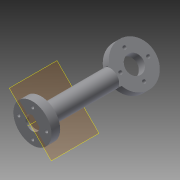
# Autodesk Inventor part: neck_v2
Saved by Autodesk Inventor 2014 (Build 180170000, 170)
## iProperties
Created: 2014-01-09
Part Number: neck_v2
Material: Générique
Document SubType Name: Modeling
Designer: helly
Density: 1 g/cm^3
Appearance: Par défaut
Author: helly
Autodesk Inventor part; units mm, degrees
ref_plane "YZ Plane" through (0, 0, 0) normal (1, 0, 0) x (0, 1, 0)
ref_plane "XZ Plane" through (0, 0, 0) normal (0, 1, 0) x (-1, 0, 0)
sketch "Esquisse1" plane through (0, 0, 0) normal (0, 1, 0) x (-1, 0, 0)
  circle A0 centre (0, 0) radius 11
  line L0 (0, 0) -> (-8, 0) construction
  circle A1 centre (-8, 0) radius 1
  circle A2 centre (0, -8) radius 1
  circle A3 centre (8, 0) radius 1
  circle A4 centre (0, 8) radius 1
  circle A5 centre (0, 0) radius 4
  dimension "d0" = 22
  dimension "d1" = 8
  dimension "d2" = 2
  dimension "d5" = 360
  dimension "d7" = 8
  constraints: 6 centre point, 5 coincident, 2 end point, 1 horizontal, 11 other
  measures "d0" diameter of A0
  measures "d1" distance of L0.start L0.end
  measures "d2" diameter of A1
  measures "d7" diameter of A5
extrude "Extrusion1" add sketch "Esquisse1" along normal blind 5
sketch "Esquisse2" plane through (0, 5, 0) normal (0, 1, 0) x (1, 0, 0)
  circle A0 centre (0, 0) radius 4 projected
extrude "Extrusion2" add sketch "Esquisse2" against normal blind 3
sketch "Esquisse3" plane through (0, 5, 0) normal (0, 1, 0) x (1, 0, 0)
  circle A0 centre (0, 0) radius 11 projected
  circle A1 centre (0, 0) radius 5
  dimension "d12" = 10
  constraints: 1 centre point, 1 coincident
  measures "d12" diameter of A1
extrude "Extrusion3" add sketch "Esquisse3" along normal blind 40 contours A1
ref_plane "Plan de construction1" through (0, 0, 0) normal (0.7071, 0, 0.7071) x (0, 1, 0)
sketch "Esquisse4" plane through (0, 0, 0) normal (0.7071, 0, 0.7071) x (0, 1, 0)
  line L0 (0, 0) -> (5, 0) construction
  line L1 (5, 0) -> (5, -5) construction
  line L2 (5, 0) -> (5, 5)
  line L3 (5, 0) -> (5, -5)
  line L4 (0, 0) -> (45, 0) construction
  line L5 (45, 0) -> (57, 0) construction
  circle A0 centre (57, 0) radius 12
  circle A1 centre (57, 0) radius 8 construction
  line L6 (0, 0) -> (45, 0) construction
  line L7 (45, 0) -> (57, 0) construction
  circle A2 centre (65, 0) radius 1
  circle A3 centre (57, 8) radius 1
  circle A4 centre (49, 0) radius 1
  circle A5 centre (57, -8) radius 1
  circle A6 centre (57, 0) radius 5
  line L8 (46.0913, 5) -> (45, 5)
  line L9 (45, 5) -> (45, 0)
  line L10 (45, -5) -> (46.0913, -5)
  line L11 (45, 0) -> (45, -5)
  dimension "d53" = 16
  dimension "d36" = 45
  dimension "d52" = 12
  dimension "d54" = 2
  dimension "d57" = 360
  dimension "d59" = 10
  constraints: 24 end point, 6 centre point, 5 perpendicular, 4 collinear, 3 coincident, 3 point on circle, 2 tangent, 1 horizontal alignment, 1 parallel, 11 other
  measures "d36" distance of L0.start L4.end
  measures "d52" distance of L4.end L5.end
  measures "d54" diameter of A2
  measures "d59" diameter of A6
extrude "Extrusion6" add sketch "Esquisse4" along normal mid plane 5
